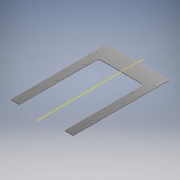
# Autodesk Inventor part: Front
Saved by Autodesk Inventor 2018 (Build 220112000, 112)
## iProperties
Created: 2017-10-08
Part Number: Front
Material: Edelstahl
Document SubType Name: Blech
Designer: jro
Density: 8 g/cm^3
Sheet Metal Rule: Standard_mm
Appearance: Halbpoliert
Mass: 436.49 g
Surface Area: 580.02 cm^2
Volume: 54.5612 cm^3
Author: jro
Autodesk Inventor part; units mm, degrees
ref_plane "YZ Plane" through (0, 0, 0) normal (1, 0, 0) x (0, 1, 0)
ref_plane "XZ Plane" through (0, 0, 0) normal (0, 1, 0) x (-1, 0, 0)
ref_plane "XY Plane" through (0, 0, 0) normal (0, 0, 1) x (1, 0, 0)
sketch "Skizze1" plane through (0, 0, 0) normal (0, 0, 1) x (1, 0, 0)
  line L0 (106.9629, 2) -> (-106.9629, 2)
  line L1 (0, -19.6018) -> (0, 5.6106)
  line L2 (0, 2) -> (81.5, 2)
  line L3 (0, 2) -> (-81.5, 2)
  line L4 (-81.5, 2) -> (-81.5, 277)
  line L5 (81.5, 2) -> (81.5, 277)
  line L6 (71.5, 287) -> (-71.5, 287)
  arc A0 (81.5, 277) -> (71.5, 287) centre (71.5, 277) ccw
  arc A1 (-71.5, 287) -> (-81.5, 277) centre (-71.5, 277) ccw
  line L7 (-81.5, 2) -> (-106.9629, 2)
  line L8 (-106.9629, 2) -> (-106.9629, 347)
  line L9 (81.5, 2) -> (106.9629, 2)
  line L10 (106.9629, 2) -> (106.9629, 347)
  line L11 (106.9629, 347) -> (-106.9629, 347)
  point P0 (0, 0)
  point P1 (-81.5, 287)
  point P2 (81.5, 287)
  point P3 (-106.9629, 347)
  dimension "d7" = 0
  dimension "d0" = 81.5
  dimension "d1" = 81.5
  dimension "PortalHoehe" = 285
  dimension "d3" = 285
  dimension "d4" = 10
  dimension "GesammtHoehe" = 345
  dimension "d6" = 345
  measures "d0" distance of L2.start L2.end
  measures "d1" distance of L2.start L3.end
  measures "PortalHoehe" distance of L3.end point (-81.5, 287)
  measures "d3" distance of L2.end point (81.5, 287)
  measures "d4" radius of A0
  measures "GesammtHoehe" distance of L0.end point (-106.963, 347)
  measures "d6" distance of L0.start point (106.963, 347)
extrude "Grobblech1" add sketch "Skizze1" along normal blind 2 contours L0 L5 A0 L6 A1 L4 L8 L11 L10
fillet "Rundung1" radius 2 2 edges at (-81.5, 2, 1) (81.5, 2, 1)
sketch "Skizze3" plane through (0, 0, 0) normal (0, 0, -1) x (-1, 0, 0)
  arc A0 (-83.5, 2) -> (-81.5, 4) centre (-83.5, 4) ccw projected
  line L0 (-81.5, 277) -> (-81.5, 4) projected
  arc A1 (-71.5, 287) -> (-81.5, 277) centre (-71.5, 277) ccw projected
  line L1 (71.5, 287) -> (-71.5, 287) projected
  arc A2 (81.5, 277) -> (71.5, 287) centre (71.5, 277) ccw projected
  line L2 (81.5, 4) -> (81.5, 277) projected
  arc A3 (81.5, 4) -> (83.5, 2) centre (83.5, 4) ccw projected
  line L3 (106.9629, 2) -> (83.5, 2) projected
  line L4 (106.9629, 347) -> (106.9629, 2) projected
  line L5 (-106.9629, 347) -> (106.9629, 347) projected
  line L6 (-106.9629, 2) -> (-106.9629, 347) projected
  line L7 (-83.5, 2) -> (-106.9629, 2) projected
  circle A4 centre (-87.5, 142) radius 2.15
  circle A5 centre (87.5, 142) radius 2.15
  circle A6 centre (-87.5, 242) radius 2.15
  circle A7 centre (87.5, 242) radius 2.15
  point P0 (0, 0)
  dimension "Durchmesser" = 4.3
  dimension "d23" = 140
  dimension "d24" = 6
  dimension "d25" = 4.3
  dimension "d26" = 6
  dimension "d27" = 140
  dimension "d30" = 4.3
  dimension "d31" = 4.3
  dimension "d32" = 6
  dimension "d33" = 6
  dimension "d34" = 100
  dimension "d35" = 100
  constraints: 4 centre point
  measures "Durchmesser" diameter of A4
  measures "d23" distance from line of L7 A4.centre
  measures "d24" distance from line of L0 A4.centre
  measures "d25" diameter of A5
  measures "d26" distance from line of L2 A5.centre
  measures "d27" distance from line of L3 A5.centre
  measures "d30" diameter of A6
  measures "d31" diameter of A7
  measures "d32" distance from line of L0 A6.centre
  measures "d33" distance from line of L2 A7.centre
  measures "d34" distance of A5.centre A7.centre
  measures "d35" distance of A4.centre A6.centre
extrude "Extrusion3" cut sketch "Skizze3" against normal through all contours A4 | A5 | A6 | A7
ref_plane "Arbeitsebene1" through (0, 2, 0) normal (-1, 0, 0) x (0, 0, 1)
sketch "Skizze4" plane through (0, 0, 0) normal (0, 0, -1) x (-1, 0, 0)
  line L0 (-106.9629, 2) -> (-106.9629, 347) projected
  line L1 (-111.9999, 2) -> (-111.9999, 339.9629)
  line L2 (106.9629, 347) -> (106.9629, 2) projected
  line L3 (111.9999, 339.9629) -> (111.9999, 2)
  line L4 (-106.9629, 2) -> (-83.5, 2) projected
  line L5 (-106.9629, 2) -> (-111.9999, 2)
  line L6 (-111.9999, 2) -> (-111.9999, 347)
  line L7 (-111.9999, 347) -> (-106.9629, 347)
  line L8 (-106.9629, 347) -> (-106.9629, 2)
  line L9 (106.9629, 2) -> (106.9629, 347) projected
  line L10 (106.9629, 2) -> (111.9999, 2)
  line L11 (111.9999, 2) -> (111.9999, 347)
  line L12 (111.9999, 347) -> (106.9629, 347)
  line L13 (106.9629, 347) -> (106.9629, 2)
  point P0 (0, 0)
  dimension "d38" = 223.9998
  dimension "d39" = 345
  constraints: 20 end point, 4 parallel, 2 horizontal, 2 perpendicular, 2 point on line, 2 vertical, 4 other
  measures "d38" distance between parallel lines of L3 L6
  measures "d39" distance between parallel lines of L12 L4
extrude "Extrusion4" add sketch "Skizze4" against normal up to surface (2 mm away)
fillet "Rundung2" radius 2 4 edges at (111.9999, 2, 1) (111.9999, 347, 1) (-111.9999, 347, 1) (-111.9999, 2, 1)
sketch "Skizze6" plane through (0, 0, 0) normal (0, 0, -1) x (-1, 0, 0)
  circle A0 centre (-101.9999, 302) radius 2.15
  circle A1 centre (-101.9999, 192) radius 2.15
  circle A2 centre (-101.9999, 82) radius 2.15
  circle A3 centre (101.9999, 82) radius 2.15
  circle A4 centre (101.9999, 192) radius 2.15
  circle A5 centre (101.9999, 302) radius 2.15
  point P0 (0, 0)
  constraints: 6 centre point, 12 other
extrude "Extrusion5" cut sketch "Skizze6" against normal through all
equation "\"d0\" = 0.5 * PortalBreite"
equation "\"d1\" = 0.5 * PortalBreite"
equation "\"d25\" = Durchmesser"
equation "\"d26\" = d24"
equation "\"d27\" = d23"
equation "\"d30\" = Durchmesser"
equation "\"d31\" = Durchmesser"
equation "\"d32\" = d24"
equation "\"d33\" = d24"
equation "\"d35\" = d34"
equation "\"d8\" = Stärke"
equation "\"d3\" = PortalHoehe"
equation "\"d6\" = GesammtHoehe"
equation "\"PortalBreite\" = 163"
equation "\"Biegeradius\" = Stärke"
equation "\"BreiteBiegungsfreistellung\" = Stärke"
equation "\"TiefeBiegungsfreistellung\" = 0.5 * Stärke"
equation "\"GrößeEckenfreistellung\" = 4 * Stärke"
equation "\"MinimalRest\" = 2 * Stärke"
equation "\"Übergangsradius\" = Biegeradius"
equation "\"JacobiRadiusGröße\" = Biegeradius"
equation "\"Abstandsgröße\" = Stärke"
equation "\"Stärke\" = 2"
